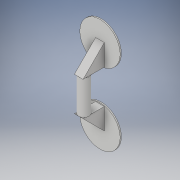
# Autodesk Inventor part: SuctionCup
Saved by Autodesk Inventor 2019 (Build 230136000, 136)
## iProperties
Created: 2019-01-19
Part Number: SuctionCup
Material: Generic
Document SubType Name: Modeling
Designer: nxgam
Density: 1 g/cm^3
Appearance: Default
Author: nxgam
Autodesk Inventor part; units mm, degrees
ref_plane "YZ Plane" through (0, 0, 0) normal (1, 0, 0) x (0, 1, 0)
ref_plane "XZ Plane" through (0, 0, 0) normal (0, 1, 0) x (-1, 0, 0)
ref_plane "XY Plane" through (0, 0, 0) normal (0, 0, 1) x (1, 0, 0)
sketch "Sketch1" plane through (0, 0, 0) normal (0, 1, 0) x (-1, 0, 0)
  circle A0 centre (0, 0) radius 14.986
  dimension "d0" = 29.972
  constraints: 1 centre point, 1 coincident
  measures "d0" diameter of A0
extrude "Extrusion1" add sketch "Sketch1" along normal mid plane 99.06
sketch "Sketch2" plane through (0, 0, 0) normal (1, 0, 0) x (0, 1, 0)
  line L0 (-49.53, 14.986) -> (-49.53, -14.986) projected
  line L1 (49.53, -14.986) -> (49.53, 14.986) projected
  line L2 (0, 14.986) -> (0, -71.9195) construction
  line L3 (49.53, 14.986) -> (49.53, -46.736)
  line L4 (49.53, -46.736) -> (111.252, -46.736)
  line L5 (111.252, -46.736) -> (49.53, 14.986)
  line L6 (-49.53, -14.986) -> (-49.53, 14.986)
  line L7 (-49.53, 14.986) -> (-49.53, -46.736)
  line L8 (-49.53, -46.736) -> (-111.252, -46.736)
  line L9 (-111.252, -46.736) -> (-49.53, 14.986)
  point P0 (0, 0)
  dimension "d3" = 61.722
  dimension "d4" = 61.722
  constraints: 16 end point, 2 symmetric about line, 2 vertical, 1 horizontal
  measures "d3" distance of L1.end L3.end
  measures "d4" distance of L3.end L4.end
extrude "Extrusion2" add sketch "Sketch2" along normal mid plane 25.4
sketch "Sketch3" plane through (12.7, 111.252, -46.736) normal (0, 0, -1) x (-1, 0, 0)
  line L0 (12.7, -111.252) -> (12.7, -6.477) construction
  circle A0 centre (12.7, -6.477) radius 58.42
  line L1 (12.7, -111.252) -> (-79.2707, -111.252) construction
  circle A1 centre (12.7, -216.027) radius 58.42
  dimension "d7" = 104.775
  dimension "d8" = 116.84
  constraints: 4 end point, 2 centre point, 1 coincident, 1 horizontal, 1 symmetric about line, 1 vertical, 1 other
  measures "d7" distance of L0.start L0.end
  measures "d8" diameter of A0
extrude "Extrusion3" add sketch "Sketch3" along normal blind 3.81
equation "\"d4\" = d3"
body "Solid1"
